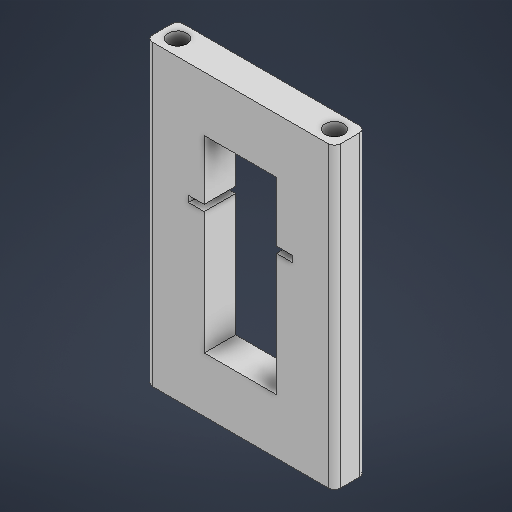
# Autodesk Inventor part: SERVO držák
Saved by Autodesk Inventor 2026 (Build 300175050, 175E)
## iProperties
Created: 2026-02-25
Part Number: SERVO držák
Material: Všeobecné
Document SubType Name: Modeling
Designer: marti
Density: 1 g/cm^3
Appearance: Výchozí
Author: marti
Autodesk Inventor part; units mm, degrees
ref_plane "YZ Plane" through (0, 0, 0) normal (1, 0, 0) x (0, 1, 0)
ref_plane "XZ Plane" through (0, 0, 0) normal (0, 1, 0) x (-1, 0, 0)
ref_plane "XY Plane" through (0, 0, 0) normal (0, 0, 1) x (1, 0, 0)
sketch "Náčrt1" plane through (0, 0, 0) normal (0, 0, 1) x (1, 0, 0)
  line L0 (30, -47.5) -> (-30, -47.5)
  line L1 (-30, -47.5) -> (-30, 47.5)
  line L2 (-30, 47.5) -> (30, 47.5)
  line L3 (30, 47.5) -> (30, -47.5)
  line L4 (30, -47.5) -> (-30, 47.5) construction
  line L5 (-30, -47.5) -> (30, 47.5) construction
  line L6 (-11.5, -30) -> (11.5, -30)
  line L7 (11.5, -30) -> (11.5, 30)
  line L8 (11.5, 30) -> (-11.5, 30)
  line L9 (-11.5, 30) -> (-11.5, -30)
  line L10 (-11.5, -30) -> (11.5, 30) construction
  line L11 (11.5, -30) -> (-11.5, 30) construction
  line L12 (0, 66.5) -> (0, -66.5) projected
  line L13 (-42, 0) -> (42, 0) projected
  point P0 (0, 0)
  point P1 (0, 0)
  dimension "d25" = 60
  dimension "d26" = 95
  dimension "d27" = 23
  dimension "d28" = 60
  constraints: 24 end point, 5 midpoint, 4 parallel, 2 horizontal, 2 perpendicular, 2 other
  measures "d25" distance of L1.end L2.end
  measures "d26" distance of L0.end L1.end
  measures "d27" distance of L8.end L7.end
  measures "d28" distance of L7.end L6.end
extrude "Vysunutí1" add sketch "Náčrt1" along normal mid plane 10 contours L0 L12 L6 L7 L13 L3 | L0 L1 L13 L9 L6 L12 | L13 L7 L8 L12 L2 L3 | L1 L2 L12 L8 L9 L13
sketch "Náčrt2" plane through (-30, 47.5, 5) normal (0, 1, 0) x (1, 0, 0)
  point P0 (5, 5)
  point P1 (55, 5)
hole "Díra1" at (-25, 47.5, 0) at (25, 47.5, 0) direction (0, -1, 0) diameter 6 end through all
fillet "Zaoblení1" radius 2 4 edges at (-30, 0, 5) (-30, 0, -5) (30, 0, -5) (30, 0, 5)
sketch "Náčrt3" plane through (0, 0, 5) normal (0, 0, 1) x (1, 0, 0)
  line L0 (11.5, 30) -> (11.5, -30) projected
  line L1 (11.5, 9) -> (16.5, 9)
  line L2 (16.5, 9) -> (16.5, 11)
  line L3 (16.5, 11) -> (11.5, 11)
  line L4 (11.5, 11) -> (11.5, 9)
  line L5 (-42, 0) -> (42, 0) projected
  line L6 (0, 66.5) -> (0, -66.5) projected
  line L7 (-11.5, 30) -> (11.5, 30) projected
  line L8 (28, 47.5) -> (-28, 47.5) projected
  line L9 (-11.5, 9) -> (-16.5, 9)
  line L10 (-16.5, 9) -> (-16.5, 11)
  line L11 (-16.5, 11) -> (-11.5, 11)
  line L12 (-11.5, 11) -> (-11.5, 9)
  point P0 (0, 0)
  point P1 (14, 11)
  point P2 (-14, 11)
  dimension "d47" = 5
  dimension "d48" = 2
  dimension "d50" = 36.5
  constraints: 16 end point, 5 symmetric about line, 2 parallel, 1 horizontal, 1 midpoint, 1 perpendicular, 1 point on line
  measures "d47" distance of L3.end L2.end
  measures "d48" distance of L2.end L1.end
  measures "d50" distance from line of L8 point (14, 11)
extrude "Vysunutí3" cut sketch "Náčrt3" against normal blind 36.5 contours L3 L2 L1 L0 | L9 L10 L11 L12
equation "\"d51\" = d50"
